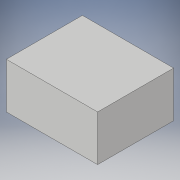
# Autodesk Inventor part: Regulator-LT1965
Saved by Autodesk Inventor 2018 (Build 220112000, 112)
## iProperties
Created: 2018-04-09
Part Number: Regulator-LT1965
Material: Generic
Document SubType Name: Modeling
Designer: bbramman
Density: 1 g/cm^3
Appearance: Default
Author: bbramman
Autodesk Inventor part; units mm, degrees
ref_plane "YZ Plane" through (0, 0, 0) normal (1, 0, 0) x (0, 1, 0)
ref_plane "XZ Plane" through (0, 0, 0) normal (0, 1, 0) x (-1, 0, 0)
ref_plane "XY Plane" through (0, 0, 0) normal (0, 0, 1) x (1, 0, 0)
sketch "Sketch1" plane through (0, 0, 0) normal (0, 1, 0) x (-1, 0, 0)
  line L0 (-4.5, 3.75) -> (4.5, 3.75)
  line L1 (4.5, 3.75) -> (4.5, -3.75)
  line L2 (4.5, -3.75) -> (-4.5, -3.75)
  line L3 (-4.5, -3.75) -> (-4.5, 3.75)
  line L4 (-4.5, 3.75) -> (4.5, -3.75) construction
  line L5 (4.5, 3.75) -> (-4.5, -3.75) construction
  point P0 (0, 0)
  dimension "d0" = 9
  dimension "d1" = 7.5
  constraints: 12 end point, 2 midpoint, 2 parallel, 1 horizontal, 1 perpendicular
  measures "d0" distance of L1.end L2.end
  measures "d1" distance of L0.end L1.end
extrude "Extrusion1" add sketch "Sketch1" along normal blind 4.5
body "Solid1"
